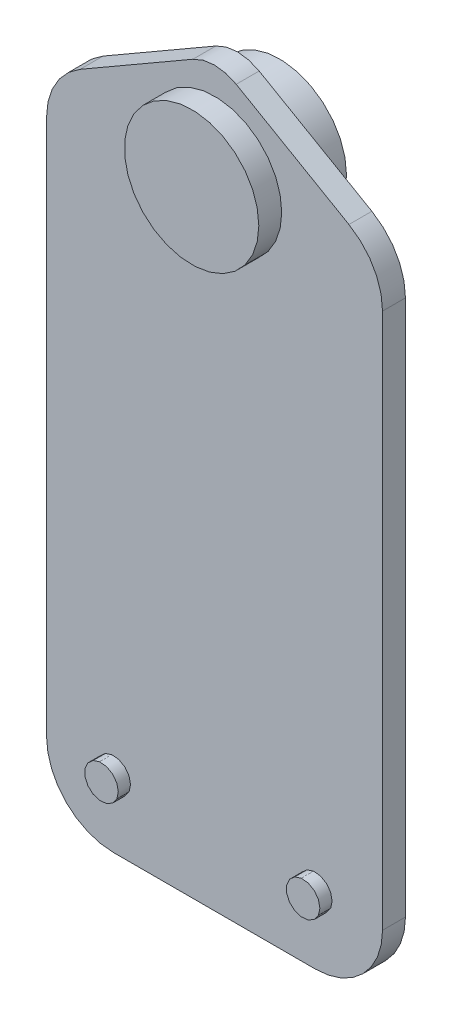
# Autodesk Inventor part: WheelHolder
Saved by Autodesk Inventor 2012 SP2 (Build 160219200, 219)
## iProperties
Created: 2013-07-20
Part Number: WheelHolder
Material: Default
Document SubType Name: Modeling
Designer: 1
Density: 1 g/cm^3
Author: 1
Autodesk Inventor part; units mm, degrees
ref_plane "YZ Plane" through (0, 0, 0) normal (1, 0, 0) x (0, 1, 0)
ref_plane "XZ Plane" through (0, 0, 0) normal (0, 1, 0) x (-1, 0, 0)
ref_plane "XY Plane" through (0, 0, 0) normal (0, 0, 1) x (1, 0, 0)
sketch "Sketch1" plane through (0, 0, 0) normal (0, 0, 1) x (1, 0, 0)
  circle A0 centre (-40, 926.5) radius 10 projected
  circle A1 centre (-40, 926.5) radius 14 projected
  line L0 (-65, 921.2927) -> (-65, 841.5)
  line L1 (-55, 831.5) -> (-40, 831.5)
  arc A2 (-60, 929.953) -> (-65, 921.2927) centre (-55, 921.2927) ccw
  arc A3 (-65, 841.5) -> (-55, 831.5) centre (-55, 841.5) ccw
  line L2 (-40, 926.5) -> (-40, 831.5) construction
  line L3 (-40, 936.5) -> (-40, 831.5) construction
  circle A4 centre (-40, 926.5) radius 10
  line L4 (-15, 921.2927) -> (-15, 841.5)
  line L5 (-25, 831.5) -> (-40, 831.5)
  arc A5 (-15, 921.2927) -> (-20, 929.953) centre (-25, 921.2927) ccw
  arc A6 (-25, 831.5) -> (-15, 841.5) centre (-25, 841.5) ccw
  line L6 (-60, 929.953) -> (-43.2258, 939.6376)
  line L7 (-36.7742, 939.6376) -> (-20, 929.953)
  arc A7 (-36.7742, 939.6376) -> (-43.2258, 939.6376) centre (-40, 934.0503) ccw
  point P0 (0, 0)
  point P1 (-40, 941.5)
  dimension "d0" = 10
  dimension "d1" = 25
  dimension "d3" = 95
  dimension "d4" = 15
  dimension "d5" = 6.4516
  dimension "d6" = 120
  dimension "d7" = 4.3301
  constraints: 16 end point, 10 point on circle, 6 symmetric about line, 6 tangent, 5 centre point, 3 point on line, 2 perpendicular, 1 collinear, 1 equal radius, 1 vertical, 3 other
  measures "d0" radius of A2
  measures "d1" distance from line of L1.end L0
  measures "d3" distance from line of L1 A0.centre
  measures "d4" distance of A0.centre point (-40, 941.5)
  measures "d5" radius of A7
  measures "d6" angle of L0 L6
  measures "d7" distance from line of L3.start L7
extrude "Extrusion1" add sketch "Sketch1" along normal blind 3.4125 contours A0 | A1 L6 A7 L7 | A1 L7 A5 L4 A6 L5 L1 A3 L0 A2 L6
sketch "Sketch2" plane through (0, 0, 3.4125) normal (0, 0, 1) x (1, 0, 0)
  circle A0 centre (-40, 926.5) radius 10 projected
  circle A1 centre (-40, 926.5) radius 10
  point P0 (0, 0)
  constraints: 1 centre point, 1 coincident, 1 concentric
extrude "Extrusion2" add sketch "Sketch2" along normal blind 3.4125 and the other way blind 9.6435
sketch "Sketch3" plane through (-40, 926.5, 6.825) normal (0, 0, 1) x (1, 0, 0)
  circle A0 centre (0, 0) radius 10 projected
  point P0 (40, -926.5)
sketch "Sketch4" plane through (0, 0, 3.4125) normal (0, 0, 1) x (1, 0, 0)
  arc A0 (-65, 841.5) -> (-55, 831.5) centre (-55, 841.5) ccw projected
  arc A1 (-25, 831.5) -> (-15, 841.5) centre (-25, 841.5) ccw projected
  circle A2 centre (-55, 841.5) radius 2.5
  circle A3 centre (-25, 841.5) radius 2.5
  point P0 (0, 0)
  dimension "d14" = 5
  constraints: 2 centre point, 2 coincident, 1 equal radius
  measures "d14" diameter of A2
extrude "Extrusion3" add sketch "Sketch4" along normal blind 1.825
body "Solid1"
